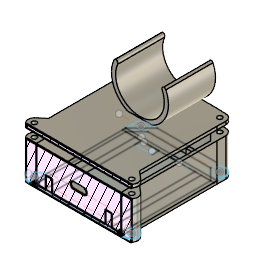
UM982 holder v4 (Autodesk Fusion 360 design; units mm, degrees)
Autodesk Fusion 360 part; units mm, degrees
note: some values were not read from the file. Chosen so that the rebuilt part matches the saved one: which face or edge a step refers to; which pieces of a blend or face edit are solid. Set by a fixed rule: which sketch regions a step uses.
sketch "Sketch1" plane through (0, 0, 0) normal (0, 0, 1) x (1, 0, 0)
  line L0 (0, 0) -> (54, 0)
  line L1 (54, 0) -> (54, 57.2)
  line L2 (54, 57.2) -> (0, 57.2) construction
  line L3 (0, 57.2) -> (0, 0)
  line L4 (32, 0) -> (22, 0)
  line L5 (22, 0) -> (22, -2)
  line L6 (22, -2) -> (32, -2)
  line L7 (32, -2) -> (32, 0)
  line L8 (54, 0) -> (56, 0)
  line L9 (0, 0) -> (-2, 0)
  line L10 (-2, 0) -> (-2, 59.2)
  line L11 (-2, 0) -> (22, 0)
  line L12 (22, 0) -> (22, -2)
  line L13 (22, -2) -> (-2, -2)
  line L14 (-2, -2) -> (-2, 0)
  line L15 (32, -2) -> (56, -2)
  line L16 (56, -2) -> (56, 0)
  line L17 (56, 0) -> (32, 0)
  line L18 (32, 0) -> (32, -2)
  line L19 (-2, 59.2) -> (56, 59.2)
  line L20 (56, 59.2) -> (56, 57.2)
  line L21 (56, 57.2) -> (-2, 57.2)
  line L22 (-2, 57.2) -> (-2, 59.2)
  line L23 (56, 57.2) -> (56, 0)
  line L24 (29, 57.2) -> (34, 57.2)
  line L25 (54, 5) -> (54, 10)
  line L26 (5, 0) -> (0, 0)
  line L27 (0, 0) -> (0, 5)
  line L28 (6, 57.2) -> (10, 57.2)
  line L29 (10, 57.2) -> (10, 0)
  line L30 (6, 0) -> (6, 57.2)
  line L31 (48, 57.2) -> (48, 0)
  line L32 (44, 57.2) -> (44, 0)
  line L33 (-2, 59.2) -> (8, 69.2)
  line L34 (-2, 59.2) -> (7.8995, 59.2) construction
  line L35 (8, 69.2) -> (46, 69.2)
  line L36 (46, 69.2) -> (56, 59.2)
  line L37 (0, 57.2) -> (7, 64.2)
  line L38 (0, 57.2) -> (11.5737, 57.2) construction
  line L39 (7, 64.2) -> (47, 64.2)
  line L40 (47, 64.2) -> (54, 57.2)
  line L41 (38.3605, 57.2) -> (38.3605, 59.2)
  line L42 (10, 57.2) -> (21, 57.2)
  line L43 (21, 57.2) -> (21, 53)
  line L44 (21, 53) -> (10, 53)
  line L45 (10, 53) -> (10, 57.2)
  circle A0 centre (19, 55) radius 0.9
  circle A1 centre (58, 3) radius 4
  line L46 (56, -2) -> (59.3831, -0.7533)
  line L47 (60.6098, 6.0314) -> (56, 10)
  circle A2 centre (52.048, 64.9527) radius 4
  line L48 (52.048, 64.9527) -> (-12, 64.9527) construction
  circle A3 centre (1.9352, 64.9527) radius 4
  line L49 (-2, 59.2) -> (-2.0646, 64.9074)
  line L50 (8, 69.2) -> (1.7743, 68.9495)
  line L51 (46, 69.2) -> (52.2092, 68.9494)
  line L52 (56, 59.2) -> (56.0478, 64.9192)
  line L53 (58, 3) -> (-8, 3) construction
  circle A4 centre (-4, 3) radius 4
  line L54 (-2, -2) -> (-5.3831, -0.7533)
  line L55 (-6.6098, 6.0314) -> (-2, 10)
  circle A5 centre (-4, 3) radius 1.5
  circle A6 centre (58, 3) radius 1.5
  circle A7 centre (52.048, 64.9527) radius 1.5
  circle A8 centre (1.9352, 64.9527) radius 1.5
  circle A9 centre (0, 0) radius 0.25
  circle A10 centre (54, 0) radius 0.25
  line L56 (-2, 10) -> (56, 10) construction
  dimension "d1" = 54
  dimension "d2" = 57.2
  dimension "d3" = 22
  dimension "d4" = 22
  dimension "d5" = 2
  dimension "d6" = 2
  dimension "d7" = 2
  dimension "d8" = 59.2
  dimension "d9" = 58
  dimension "d10" = 2
  dimension "d11" = 6
  dimension "d12" = 4
  dimension "d13" = 6
  dimension "d14" = 4
  dimension "d21" = 45
  dimension "d22" = 45
  dimension "d23" = 10
  dimension "d25" = 45
  dimension "d26" = 135
  dimension "d27" = 5
  dimension "d52" = 1.8
  dimension "d53" = 9
  dimension "d54" = 2
  dimension "d55" = 8
  dimension "d56" = 8
  dimension "d57" = 8
  dimension "d58" = 8
  dimension "d60" = 3
  dimension "d61" = 3
  dimension "d63" = 3
  dimension "d64" = 3
  dimension "d65" = 0.5
  dimension "d66" = 0.5
  dimension "d75" = 4
  dimension "d76" = 4
  constraint horizontal L0
  constraint vertical L1
  constraint horizontal L2
  constraint vertical L3
  constraint coincident L0.start L3.end
  constraint horizontal L4
  constraint vertical L5
  constraint horizontal L6
  constraint vertical L7
  constraint coincident L0 L4.start
  constraint perpendicular L1 L8
  constraint perpendicular L3 L9
  constraint perpendicular L2 L10
  constraint horizontal L11
  constraint vertical L12
  constraint horizontal L13
  constraint vertical L14
  constraint horizontal L15
  constraint vertical L16
  constraint horizontal L17
  constraint vertical L18
  constraint horizontal L19
  constraint vertical L20
  constraint horizontal L21
  constraint vertical L22
  constraint horizontal L24
  constraint coincident L2 L24.start
  constraint vertical L25
  constraint coincident L1 L25.end
  constraint horizontal L26
  constraint vertical L27
  constraint coincident L11 L26.start
  constraint coincident L3 L27.end
  constraint horizontal L28
  constraint vertical L29
  constraint vertical L30
  constraint coincident L21 L28.start
  constraint coincident L0 L30.start
  constraint midpoint L11 L29.end
  constraint coincident L2 L31.start
  constraint coincident L17 L31.end
  constraint coincident L2 L32.start
  constraint coincident L17 L32.end
  constraint horizontal L34
  constraint perpendicular L22 L35
  constraint horizontal L38
  constraint parallel L2 L39
  constraint coincident L21 L41.start
  constraint coincident L19 L41.end
  constraint perpendicular L19 L41
  constraint horizontal L42
  constraint vertical L43
  constraint horizontal L44
  constraint vertical L45
  constraint coincident A1 L46.end
  constraint tangent A1 L46
  constraint coincident A1 L47.start
  constraint coincident L23 L47.end
  constraint coincident A2.centre L48.start
  constraint parallel L39 L48
  constraint coincident L48 A3.centre
  constraint coincident A3 L49.end
  constraint tangent A3 L49
  constraint coincident A3 L50.end
  constraint tangent A3 L50
  constraint coincident A2 L51.end
  constraint tangent A2 L51
  constraint coincident A2 L52.end
  constraint tangent A2 L52
  constraint coincident A1.centre L53.start
  constraint perpendicular L10 L53
  constraint coincident L53 A4.centre
  constraint tangent L27 A4
  constraint coincident A4 L54.end
  constraint tangent A4 L54
  constraint coincident A4 L55.start
  constraint coincident L10 L55.end
  constraint tangent A4 L55
  constraint concentric A4 A5
  constraint concentric A1 A6
  constraint concentric A2 A7
  constraint concentric A3 A8
  constraint coincident L0.end L1.start
  constraint perpendicular L23 L56
  constraint tangent A1 L47
  measures "d1" distance of L0.start L0.end
  measures "d2" distance of L0.end L1.end
  measures "d3" distance of L0.end L7
  measures "d4" distance of L0.start L5
  measures "d5" distance of L4.start L6.end
  measures "d6" distance of L0.end L8.end
  measures "d7" distance of L0.start L9.end
  measures "d8" distance of L9.end L10.end
  measures "d9" distance of L10.end L19.end
  measures "d10" distance of L19 L21
  measures "d11" distance of L3 L30
  measures "d12" distance of L29 L30
  measures "d13" distance of L1 L31
  measures "d14" distance of L31 L32
  measures "d21" angle of L33 L34
  measures "d22" angle of L35 L36
  measures "d23" distance of L19 L35
  measures "d25" angle of L37 L38
  measures "d26" angle of L39 L40
  measures "d27" distance of L35 L39
  measures "d52" diameter of A0
  measures "d53" distance of L29 A0.centre
  measures "d54" distance of L43 A0.centre
  measures "d55" diameter of A1
  measures "d56" diameter of A2
  measures "d57" diameter of A3
  measures "d58" diameter of A4
  measures "d60" diameter of A8
  measures "d61" diameter of A6
  measures "d63" diameter of A7
  measures "d64" diameter of A5
  measures "d65" diameter of A9
  measures "d66" diameter of A10
  measures "d75" distance of L3 A4.centre
  measures "d76" distance of L1 A1.centre
extrude "Extrude1" add sketch "Sketch1" against normal blind 2 contours L0 L3 L11 L26 L27 A9 | L3 L9 L11 L27 A9 | L0 L9 L11 L26 A9 | L0 L3 L11 L21 L26 L27 L30 A9 | L0 L5 L9 L11 L12 L13 L14 L26 A4 A9 | L3 L9 L11 L27 A4 A9 | L3 L10 L21 L27 A4 | L9 L10 L11 A4 | L9 L11 L14 A4 | L0 L11 L21 L28 L29 L30 L45 | L10 A4 L55 | L10 L14 A4 | L14 A4 L54 | L0 L4 L11 L17 L21 L24 L29 L32 L43 L44 | L19 L21 L24 L28 L37 L41 L42 | L10 L19 L21 L22 L37 | L0 L4 L5 L6 L7 L12 L18 | L21 L29 L42 L43 L44 L45 | L19 L37 L39 L40 | L19 L33 L35 L36 L37 L39 L40 A2 A3 | L0 L7 L8 L15 L16 L17 L18 A1 A10 | L33 A3 L49 | L19 L21 L40 L41 | L0 L17 L21 L31 L32 | L33 A3 A8 | L33 A3 A8 | L19 L20 L21 L40 | L16 A1 L46 | L0 L1 L17 L21 L25 L31 A10 | L33 A8 | L33 A8 | L33 A3 L50 | L36 A2 L52 | L1 L21 L23 L25 A1 | L8 L16 L17 A1 | L16 L23 A1 | L0 L1 L17 A10 | L0 L8 L17 A10 | L36 A2 A7 | L36 A2 A7 | L8 L17 L23 A1 | L1 L8 L17 A1 A10 | L1 L8 L17 A10 | L36 A2 L51 | L23 A1 L47 | L36 A7 | L36 A7 | A0 | A5 | A6 makes body 1
extrude "Extrude2" add sketch "Sketch1" along normal blind 8 contours L0 L11 L21 L28 L29 L30 L45 | L0 L17 L21 L31 L32 bodies 1
extrude "Extrude3" add sketch "Sketch1" along normal blind 22 contours L3 L9 L11 L27 A9 | L0 L9 L11 L26 A9 | L0 L5 L9 L11 L12 L13 L14 L26 A4 A9 | L3 L9 L11 L27 A4 A9 | L3 L10 L21 L27 A4 | L9 L10 L11 A4 | L9 L11 L14 A4 | L10 A4 L55 | L10 L14 A4 | L14 A4 L54 | L10 L19 L21 L22 L37 | L0 L4 L5 L6 L7 L12 L18 | L19 L33 L35 L36 L37 L39 L40 A2 A3 | L0 L7 L8 L15 L16 L17 L18 A1 A10 | L33 A3 L49 | L33 A3 A8 | L33 A3 A8 | L19 L20 L21 L40 | L16 A1 L46 | L33 A8 | L33 A3 L50 | L36 A2 L52 | L1 L21 L23 L25 A1 | L8 L16 L17 A1 | L16 L23 A1 | L0 L8 L17 A10 | L36 A2 A7 | L36 A2 A7 | L8 L17 L23 A1 | L1 L8 L17 A1 A10 | L1 L8 L17 A10 | L36 A2 L51 | L23 A1 L47 | L36 A7 picked at (3.0055, 64.1618) picked at (51.268, 63.8859) bodies 1
extrude "Extrude4" add sketch "Sketch1" along normal blind 10 contours L19 L21 L40 L41 bodies 1
sketch "Sketch2" plane through (0, 64.2, 0) normal (0, -1, 0) x (1, 0, 0)
  line L0 (7, 0) -> (47, 0)
  line L1 (47, 0) -> (47, 22)
  line L2 (47, 22) -> (7, 22)
  line L3 (7, 22) -> (7, 0)
  circle A0 centre (15, 15) radius 3.25
  line L4 (20.65, 18.262) -> (15, 21.5241)
  line L5 (15, 21.5241) -> (9.35, 18.262)
  line L6 (9.35, 18.262) -> (9.35, 11.738)
  line L7 (9.35, 11.738) -> (15, 8.4759)
  line L8 (15, 8.4759) -> (20.65, 11.738)
  line L9 (20.65, 11.738) -> (20.65, 18.262)
  circle A1 centre (39, 15) radius 3.25
  line L10 (44.67, 18.2736) -> (39, 21.5472)
  line L11 (39, 21.5472) -> (33.33, 18.2736)
  line L12 (33.33, 18.2736) -> (33.33, 11.7264)
  line L13 (33.33, 11.7264) -> (39, 8.4528)
  line L14 (39, 8.4528) -> (44.67, 11.7264)
  line L15 (44.67, 11.7264) -> (44.67, 18.2736)
  point P0 (15, 15)
  point P1 (39, 15)
  dimension "d30" = 6.5
  dimension "d31" = 5.65
  dimension "d32" = 7
  dimension "d33" = 6.5
  dimension "d34" = 8
  dimension "d35" = 8
  dimension "d36" = 5.67
  constraint coincident P0 A0.centre
  constraint coincident P1 A1.centre
  measures "d30" diameter of A0
  measures "d31" distance of P0 L9
  measures "d32" distance of L2 P0
  measures "d33" diameter of A1
  measures "d34" distance of L3 P0
  measures "d35" distance of L1 P1
  measures "d36" distance of P1 L15
extrude "Extrude5" cut sketch "Sketch2" against normal blind 2.5 contours L4 L5 L6 L7 L8 L9 bodies 1
extrude "Extrude6" cut 1 faces at (15.491, 64.2, 16.317) along direction (0, 1, 0) blind 12 on bodies 1 bodies 1
sketch "Sketch3" plane through (0, -2, 0) normal (0, -1, 0) x (1, 0, 0)
  line L0 (-2, -2) -> (56, -2)
  line L1 (56, 22) -> (-2, 22)
  line L2 (22, 0) -> (22, 22) construction
  line L3 (32, 0) -> (32, 22) construction
  line L4 (-17.1, 7.1) -> (-4.55, 7.1) construction
  arc A0 (-10.55, 7.1) -> (-12.05, 5.6) centre (-10.55, 5.6) ccw
  arc A1 (-12.05, 4.9) -> (-10.55, 3.4) centre (-10.55, 4.9) ccw
  line L5 (-12.05, 4.9) -> (-12.05, 5.6)
  line L6 (-3.05, 5.6) -> (-3.05, 4.9)
  arc A2 (-3.05, 5.6) -> (-4.55, 7.1) centre (-4.55, 5.6) ccw
  arc A3 (-4.55, 3.4) -> (-3.05, 4.9) centre (-4.55, 4.9) ccw
  line L7 (2, 3.4) -> (-17.1, 3.4) construction
  line L8 (30.5, 9.3) -> (23.5, 9.3)
  line L9 (22, 10.8) -> (22, 11.65)
  line L10 (23.5, 13.15) -> (30.5, 13.15)
  line L11 (32, 11.65) -> (32, 10.8)
  line L12 (-2, 0) -> (56, 0)
  arc A4 (23.5, 13.15) -> (22, 11.65) centre (23.5, 11.65) ccw
  arc A5 (32, 11.65) -> (30.5, 13.15) centre (30.5, 11.65) ccw
  arc A6 (22, 10.8) -> (23.5, 9.3) centre (23.5, 10.8) ccw
  arc A7 (30.5, 9.3) -> (32, 10.8) centre (30.5, 10.8) ccw
  line L13 (22, 0) -> (32, 0)
  line L14 (-2, 22) -> (-2, -2)
  line L15 (56, -2) -> (56, 22)
  point P0 (22, 9.3)
  point P1 (22, 13.15)
  point P2 (32, 13.15)
  dimension "d41" = 9
  dimension "d42" = 1.5
  dimension "d45" = 3.85
  dimension "d46" = 10
  dimension "d47" = 1.5
  dimension "d48" = 9.3
  dimension "d51" = 3.85
  constraint coincident L1 L2.end
  constraint perpendicular L1 L2
  constraint coincident L1 L3.end
  constraint perpendicular L1 L3
  constraint vertical L6
  constraint vertical L5
  constraint tangent L6 A2
  constraint tangent L4 A2
  constraint tangent L6 A3
  constraint equal A2 A3
  constraint tangent A0 L5
  constraint equal A0 A2
  constraint tangent A1 L5
  constraint equal A1 A2
  constraint horizontal L8
  constraint vertical L9
  constraint horizontal L10
  constraint vertical L11
  constraint coincident L2 P1
  constraint coincident P1 L10
  constraint coincident P1 L9
  constraint tangent L10 A4
  constraint tangent L9 A4
  constraint coincident P2 L10
  constraint coincident P2 L11
  constraint tangent L10 A5
  constraint tangent L11 A5
  constraint equal A4 A5
  constraint coincident P0 L8
  constraint coincident P0 L9
  constraint tangent L8 A6
  constraint tangent L9 A6
  constraint equal A4 A6
  constraint tangent L8 A7
  constraint tangent L11 A7
  constraint equal A4 A7
  measures "d41" distance of L5 L6
  measures "d42" radius of A2
  measures "d45" distance of P0 P1
  measures "d46" distance of P1 P2
  measures "d47" radius of A4
  measures "d48" distance of L8 L13
  measures "d51" distance of L8 L10
extrude "Extrude7" cut sketch "Sketch3" against normal blind 9 contours L8 L9 L10 L11 A4 A5 A6 A7 bodies 1
extrude "Extrude8" add sketch "Sketch1" along normal blind 2 separate body contours L0 L3 L11 L26 L27 A9 | L3 L9 L11 L27 A9 | L0 L9 L11 L26 A9 | L0 L3 L11 L21 L26 L27 L30 A9 | L0 L5 L9 L11 L12 L13 L14 L26 A4 A9 | L3 L9 L11 L27 A4 A9 | L3 L10 L21 L27 A4 | L9 L10 L11 A4 | L9 L11 L14 A4 | L0 L11 L21 L28 L29 L30 L45 | L10 A4 L55 | L10 L14 A4 | L14 A4 L54 | L0 L4 L11 L17 L21 L24 L29 L32 L43 L44 | L19 L21 L24 L28 L37 L41 L42 | L10 L19 L21 L22 L37 | L0 L4 L5 L6 L7 L12 L18 | L21 L29 L42 L43 L44 L45 | L19 L37 L39 L40 | L19 L33 L35 L36 L37 L39 L40 A2 A3 | L0 L7 L8 L15 L16 L17 L18 A1 A10 | L33 A3 L49 | L19 L21 L40 L41 | L0 L17 L21 L31 L32 | L33 A3 A8 | L33 A3 A8 | L19 L20 L21 L40 | L16 A1 L46 | L0 L1 L17 L21 L25 L31 A10 | L33 A8 | L33 A3 L50 | L36 A2 L52 | L1 L21 L23 L25 A1 | L8 L16 L17 A1 | L16 L23 A1 | L0 L1 L17 A10 | L0 L8 L17 A10 | L36 A2 A7 | L36 A2 A7 | L8 L17 L23 A1 | L1 L8 L17 A1 A10 | L1 L8 L17 A10 | L36 A2 L51 | L23 A1 L47 | L36 A7 | A0 picked at (3.0055, 64.1618) picked at (51.268, 63.8859) makes body 2
sketch "Sketch4" plane through (0, 69.2, 0) normal (0, 1, 0) x (-1, 0, 0)
  line L0 (-46, 0) -> (-8, 0)
  line L1 (-8, 0) -> (-8, 2)
  line L2 (-8, 2) -> (-46, 2)
  line L3 (-46, 2) -> (-46, 0)
  line L4 (-27, 0) -> (-27, -16.3413) construction
  circle A0 centre (-27, -16.3413) radius 15.5
  line L5 (-13.9556, -24.7135) -> (-40.0444, -24.7135)
  circle A1 centre (-27, -16.3413) radius 18.1516
  line L6 (-40.0444, -24.7135) -> (-43.1055, -24.7135) construction
  line L7 (-13.9556, -24.7135) -> (-10.8945, -24.7135)
  line L8 (-40.0444, -24.7135) -> (-43.1055, -24.7135)
  dimension "d69" = 31
  constraint midpoint L0 L4.start
  constraint perpendicular L0 L4
  constraint coincident L4.end A0.centre
  constraint coincident A0 L5.start
  constraint coincident A0 L5.end
  constraint perpendicular L4 L5
  constraint concentric A0 A1
  constraint coincident A1 L6.end
  constraint parallel L5 L6
  constraint coincident A1 L7.end
  constraint parallel L5 L7
  measures "d69" diameter of A0
extrude "Extrude9" add sketch "Sketch4" against normal blind 30 contours L0 A0 A1 L7 L8 bodies 2
fillet "Fillet1" radius 1.5 4 edges at (40.0444, 54.2, -24.7135) (43.1055, 54.2, -24.7135) (10.8945, 54.2, -24.7135) (13.9556, 54.2, -24.7135) on bodies 2
move_body "Move1" bodies 2 to x (1, 0, 0) y (0, 1, 0) z (0, 0, 1) at (0, 0, -30)
move_body "Move2" bodies 2 to x (-1, 0, 0) y (0, 1, 0) z (0, 0, -1) at (-4, 0, -60)
move_body "Move3" bodies 2 to x (1, 0, 0) y (0, 1, 0) z (0, 0, 1) at (58, 0, 60)
equation "d8 = d2 + 2 mm"
equation "d58 = d55"
equation "d60 = d61"
equation "d63 = d61"
equation "d64 = d61"
